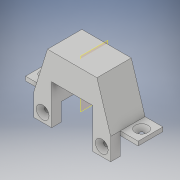
# Autodesk Inventor part: buttonHolder
Saved by Autodesk Inventor 2019 (Build 230136000, 136)
## iProperties
Created: 2019-08-23
Part Number: buttonHolder
Material: Generic
Document SubType Name: Modeling
Designer: fablab
Density: 1 g/cm^3
Appearance: Default
Author: fablab
Autodesk Inventor part; units mm, degrees
ref_plane "YZ Plane" through (0, 0, 0) normal (1, 0, 0) x (0, 1, 0)
ref_plane "XZ Plane" through (0, 0, 0) normal (0, 1, 0) x (-1, 0, 0)
ref_plane "XY Plane" through (0, 0, 0) normal (0, 0, 1) x (1, 0, 0)
sketch "Sketch1" plane through (0, 0, 0) normal (0, 1, 0) x (-1, 0, 0)
  line L0 (0, 0) -> (-30, 0)
  line L1 (-30, 0) -> (-30, -10.6)
  line L2 (-30, -10.6) -> (0, -10.6)
  line L3 (0, -10.6) -> (0, 0)
  line L4 (0, -10.6) -> (1.1, -10.6)
  line L5 (1.1, -10.6) -> (1.1, -18)
  line L6 (1.1, -18) -> (0, -18)
  line L7 (0, -18) -> (0, -10.6)
  line L8 (-30, -10.6) -> (-31.1, -10.6)
  line L9 (-31.1, -10.6) -> (-31.1, -18)
  line L10 (-31.1, -18) -> (-30, -18)
  line L11 (-30, -18) -> (-30, -10.6)
  line L12 (0, -18) -> (-30, -18)
  dimension "d0" = 30
  dimension "d1" = 10.6
  dimension "d2" = 1.1
  dimension "d3" = 1.1
  dimension "d4" = 7.4
  dimension "d5" = 7.4
  constraints: 26 end point, 6 parallel, 3 horizontal, 3 perpendicular
  measures "d0" distance of L2.end L1.end
  measures "d1" distance of L1.end L0.end
  measures "d2" distance of L5.end L6.end
  measures "d3" distance of L10.end L9.end
  measures "d4" distance of L8.end L9.end
  measures "d5" distance of L4.end L5.end
extrude "Extrusion1" add sketch "Sketch1" along normal blind 3
sketch "Sketch2" plane through (30, 0, 0) normal (1, 0, 0) x (0, 0, -1)
  point P0 (0, 0)
sketch "Sketch3" plane through (30, 0, 0) normal (1, 0, 0) x (0, 0, -1)
  line L0 (0, 0) -> (10.6, 0) projected
  line L1 (0, 0) -> (0, -30)
  line L2 (0, -30) -> (10.6, -30)
  line L3 (10.6, 0) -> (10.6, -30)
  line L4 (10.6, 0) -> (0, 0) projected
  line L5 (0, 0) -> (10.6, 0)
  dimension "d8" = 30
  constraints: 8 end point, 2 vertical, 1 collinear, 1 perpendicular
  measures "d8" distance of L0.start L1.end
sketch "Sketch4" plane through (31.1, 0, -10.6) normal (1, 0, 0) x (0, 0, -1)
  line L0 (0, 0) -> (7.4, 0) projected
  line L1 (7.4, 0) -> (7.4, -14)
  line L2 (7.4, -14) -> (0, -14)
  line L3 (0, -14) -> (0, 0)
  line L4 (0, 0) -> (7.4, 0)
  point P0 (-10.6, 0)
  dimension "d9" = 14
  constraints: 8 end point, 2 perpendicular, 1 collinear, 1 vertical
  measures "d9" distance of L0.end L1.end
extrude "Extrusion2" add sketch "Sketch3" along normal blind 3
extrude "Extrusion3" add sketch "Sketch4" along normal blind 3
sketch "Sketch5" plane through (31.1, -14, -18) normal (0, -1, 0) x (1, 0, 0)
  line L0 (1.9, 7.4) -> (1.9, 18) projected
  line L1 (1.9, 7.4) -> (1.9, 0)
  line L2 (0, 0) -> (3, 0) projected
  line L3 (-1.1, 18) -> (-1.1, 7.4) projected
  line L4 (-1.1, 7.4) -> (-1.1, 0)
  line L5 (0, 0) -> (-32.2, 0) projected
  line L6 (-1.1, 7.4) -> (1.9, 7.4) projected
  line L7 (1.9, 7.4) -> (-1.1, 7.4)
  point P0 (-31.1, 18)
  constraints: 6 end point, 2 point on line, 1 horizontal, 1 parallel, 1 vertical
extrude "Extrusion4" add sketch "Sketch5" along normal blind 16
sketch "Sketch6" plane through (30, 0, 0) normal (0, 1, 0) x (1, 0, 0)
  line L0 (1.1, 10.6) -> (1.1, 18) projected
  line L1 (1.1, 10.6) -> (1.1, 0)
  line L2 (0, 0) -> (3, 0) projected
  line L3 (1.1, 0) -> (0, 0)
  line L4 (0, 0) -> (0, 10.6)
  line L5 (0, 0) -> (0, 18) projected
  line L6 (0, 10.6) -> (1.1, 10.6) projected
  line L7 (1.1, 10.6) -> (0, 10.6)
  point P0 (-30, 0)
  constraints: 8 end point, 2 collinear, 1 point on line, 1 vertical
extrude "Extrusion5" add sketch "Sketch6" along normal blind 3
sketch "Sketch7" plane through (31.1, 3, 0) normal (1, 0, 0) x (0, 0, -1)
  point P0 (0, -3)
sketch "Sketch8" plane through (31.1, 0, 0) normal (0, 1, 0) x (1, 0, 0)
  line L0 (0, 0) -> (1.9, 0) projected
  line L1 (0, 0) -> (0, 18) projected
  line L2 (1.9, 0) -> (0, 0)
  line L3 (0, 0) -> (0, 18)
  line L4 (0, 18) -> (1.9, 18)
  line L5 (1.9, 18) -> (1.9, 0)
  point P0 (-31.1, 0)
  constraints: 8 end point, 2 parallel, 1 horizontal, 1 perpendicular
extrude "Extrusion6" add sketch "Sketch8" along normal up to surface (3 mm away)
sketch "Sketch9" plane through (33, -14, -10.6) normal (0, 0, 1) x (1, 0, 0)
  line L0 (0, 0) -> (0, 14) projected
  line L1 (0, 0) -> (1.1, 0) projected
  line L2 (1.1, 14) -> (1.1, 0) projected
  line L3 (0, 14) -> (1.1, 14) projected
  line L4 (0, 0) -> (0, 14) projected
  line L5 (0, 14) -> (1.1, 14)
  line L6 (1.1, 14) -> (1.1, 0)
  line L7 (1.1, 0) -> (0, 0)
  line L8 (0, 0) -> (0, 14)
  point P0 (-33, 14)
  constraints: 8 end point, 2 parallel, 1 horizontal, 1 perpendicular
extrude "Extrusion7" cut sketch "Sketch9" against normal blind 2000
sketch "Sketch10" plane through (33, 0, 0) normal (1, 0, 0) x (0, 0, -1)
  line L0 (0, -30) -> (0, 3) projected
  line L1 (0, -30) -> (18, -30)
  line L2 (18, -30) -> (18, -27)
  line L3 (18, -27) -> (0, -27)
  line L4 (0, -27) -> (0, -30)
  point P0 (0, 0)
  point P1 (0, 1.1)
  dimension "d25" = 18
  dimension "d26" = 3
  constraints: 8 end point, 2 parallel, 1 horizontal, 1 perpendicular
  measures "d25" distance of L3.end L2.end
  measures "d26" distance of L2.end L1.end
extrude "Extrusion8" add sketch "Sketch10" along normal blind 14
sketch "Sketch12" plane through (0, 3, 0) normal (0, 1, 0) x (1, 0, 0)
  line L0 (0, 10.6) -> (0, 0) projected
  line L1 (15, 0) -> (15, 18)
  point P0 (30, 10.6)
  point P1 (31.1, 10.6)
  point P2 (30, 0)
  constraints: 2 end point, 1 vertical
ref_plane "Work Plane1" through (15, 0, -10.6) normal (-1, 0, 0) x (0, 0, 1)
mirror "Mirror1" about plane through (15, 0, -10.6) normal (-1, 0, 0) of "Extrusion2", "Extrusion3", "Extrusion4", "Extrusion5", "Extrusion6", "Extrusion7", "Extrusion8"
sketch "Sketch13" plane through (30, -30, 0) normal (0, 0, 1) x (1, 0, 0)
  line L0 (-33, 33) -> (3, 33) projected
  line L1 (-30, 30) -> (0, 30)
  line L2 (0, 30) -> (0, 33)
  line L3 (0, 33) -> (-30, 33)
  line L4 (-30, 33) -> (-30, 30)
  point P0 (-31.1, 33)
  point P1 (1.1, 33)
  dimension "d36" = 30
  constraints: 8 end point, 2 parallel, 1 horizontal, 1 perpendicular, 1 point on line
  measures "d36" distance of L3.end L2.end
extrude "Extrusion10" add sketch "Sketch13" along normal blind 7
sketch "Sketch14" plane through (0, 0, 0) normal (0, -1, 0) x (1, 0, 0)
  line L0 (0, 0) -> (0, 7) projected
  line L1 (30, 0) -> (30, -10.6) projected
  line L2 (0, 7) -> (30, 7)
  line L3 (30, 7) -> (30, 0)
  line L4 (30, 0) -> (0, 0)
  line L5 (0, 0) -> (0, 7)
  constraints: 8 end point, 2 parallel, 1 horizontal, 1 perpendicular
extrude "Extrusion11" add sketch "Sketch14" along normal blind 14
sketch "Sketch16" plane through (0, 3, 0) normal (0, 1, 0) x (1, 0, 0)
  line L0 (30, -7) -> (0, -7) projected
  line L1 (-3, 18) -> (33, 18) projected
  line L2 (30, -7) -> (0, -7)
  line L3 (0, -7) -> (0, 18)
  line L4 (0, 18) -> (30, 18)
  line L5 (30, 18) -> (30, -7)
  line L6 (33, 18) -> (31.1, 18) projected
  line L7 (31.1, 18) -> (30, 18)
  line L8 (30, 18) -> (30, 0)
  line L9 (30, 0) -> (31.1, 0)
  line L10 (0, 0) -> (0, 18) projected
  line L11 (0, 18) -> (-1.1, 18)
  line L12 (-1.1, 0) -> (0, 0)
  line L13 (0, 0) -> (0, 18)
  line L14 (31.1, 18) -> (33, 18)
  line L15 (33, 0) -> (31.1, 0)
  line L16 (33, 0) -> (30, 0) projected
  line L17 (31.1, 18) -> (-1.1, 18) projected
  line L18 (-3, 18) -> (-17, 18) projected
  line L19 (-1.1, 18) -> (-3, 18)
  line L20 (-3, 18) -> (-3, 0) projected
  line L21 (-3, 18) -> (-3, 0)
  line L22 (-3, 0) -> (-1.1, 0)
  line L23 (0, 0) -> (-3, 0) projected
  line L24 (33, 18) -> (33, 0) projected
  line L25 (33, 18) -> (33, 0)
  constraints: 32 end point, 5 collinear, 4 horizontal, 4 parallel, 2 perpendicular, 1 point on line
extrude "Extrusion13" add sketch "Sketch16" along normal blind 2
sketch "Sketch17" plane through (30, -30, 0) normal (0, 0, 1) x (1, 0, 0)
  line L0 (0, 35) -> (3, 35) projected
  line L1 (3, 35) -> (0, 35)
  line L2 (0, 35) -> (0, 0)
  line L3 (0, 0) -> (3, 0)
  line L4 (3, 0) -> (3, 35)
  line L5 (0, 0) -> (17, 0) projected
  line L6 (0, 0) -> (13, 0)
  line L7 (13, 0) -> (13, -13.0001)
  line L8 (13, -13.0001) -> (0, -13.0001)
  line L9 (0, -13.0001) -> (0, 0)
  point P0 (-30, 30)
  dimension "d45" = 13
  constraints: 16 end point, 4 parallel, 2 horizontal, 2 perpendicular
  measures "d45" distance of L7.end L8.end
extrude "Extrusion14" add sketch "Sketch17" along normal blind 7 contours L0 L4 L3 L2
sketch "Sketch18" plane through (33, -30, 0) normal (0, 0, 1) x (1, 0, 0)
  line L0 (-3, 16) -> (-3, 0) projected
  line L1 (-3, 0) -> (10, 0)
  line L2 (10, 0) -> (10, -13)
  line L3 (10, -13) -> (-3, -13)
  line L4 (-3, -13) -> (-3, 0)
  point P0 (-33, 30)
  dimension "d48" = 13
  dimension "d49" = 13
  constraints: 8 end point, 2 parallel, 1 horizontal, 1 perpendicular
  measures "d48" distance of L2.end L3.end
  measures "d49" distance of L1.end L2.end
extrude "Extrusion15" add sketch "Sketch18" along normal blind 7
sketch "Sketch19" plane through (33, -30, 0) normal (0, 1, 0) x (1, 0, 0)
  line L0 (10, 0) -> (10, -7) projected
  line L1 (10, -7) -> (0, -7) projected
  line L2 (10, 0) -> (0, 0)
  line L3 (0, 0) -> (0, -7)
  line L4 (0, -7) -> (10, -7)
  line L5 (10, -7) -> (10, 0)
  point P0 (-33, 0)
  constraints: 8 end point, 2 parallel, 1 horizontal, 1 perpendicular
sketch "Sketch20" plane through (30, -30, 7) normal (0, 0, 1) x (1, 0, 0)
  line L0 (13, -13) -> (13, 0) projected
  line L1 (13, -6.5) -> (0, -6.5) construction
  line L2 (0, -13) -> (0, 0) projected
  line L3 (3, 0) -> (13, 0) projected
  line L4 (6.5, 0) -> (6.5, -6.5) construction
  circle A0 centre (6.5, -6.5) radius 1.65
  point P0 (-30, 30)
  dimension "d52" = 3.3
  constraints: 4 end point, 3 midpoint, 1 centre point, 1 coincident, 1 point on line
  measures "d52" diameter of A0
extrude "Extrusion16" cut sketch "Sketch20" against normal blind 7
chamfer "Chamfer3" distance 3 angle 45 1 edges at (34.85, -36.5, 7)
extrude "Extrusion17" add sketch "Sketch19" along normal blind 3
sketch "Sketch21" plane through (33, -27, -18) normal (0, 1, 0) x (1, 0, 0)
  line L0 (14, 0) -> (14, -18) projected
  line L1 (14, 0) -> (23, 0)
  line L2 (23, 0) -> (23, -18)
  line L3 (23, -18) -> (14, -18)
  line L4 (14, -18) -> (14, 0)
  point P0 (-33, -18)
  dimension "d60" = 9
  constraints: 8 end point, 2 parallel, 1 horizontal, 1 perpendicular
  measures "d60" distance of L2.end L3.end
extrude "Extrusion18" add sketch "Sketch21" against normal blind 3
sketch "Sketch22" plane through (33, -27, 7) normal (0, 1, 0) x (1, 0, 0)
  line L0 (10, 7) -> (23, 7) projected
  line L1 (16.5, 7) -> (16.5, 25) construction
  line L2 (0, 25) -> (23, 25) projected
  line L3 (23, 25) -> (23, 7) projected
  line L4 (23, 16) -> (16.5, 16) construction
  circle A0 centre (16.5, 16) radius 1.65
  point P0 (-33, 7)
  dimension "d63" = 3.3
  constraints: 4 end point, 3 midpoint, 1 centre point, 1 coincident, 1 point on line, 1 vertical
  measures "d63" diameter of A0
extrude "Extrusion19" cut sketch "Sketch22" against normal blind 3
chamfer "Chamfer4" distance 3 angle 45 1 edges at (47.85, -27, -9)
sketch "Sketch24" plane through (30, -30, 7) normal (0, 0, 1) x (1, 0, 0)
  line L0 (1.1, 30) -> (1.1, 16) projected
  line L1 (-30, 35) -> (3, 35) projected
  line L2 (-30, 16) -> (-30, 35) projected
  line L3 (0, 16) -> (-30, 16) projected
  line L4 (0, 16) -> (0, -13) projected
  line L5 (0, -13) -> (13, -13) projected
  line L6 (13, -13) -> (13, 3) projected
  line L7 (3, 3) -> (13, 3) projected
  line L8 (3, 3) -> (3, 35) projected
  circle A0 centre (6.5, -6.5) radius 4.65 projected
  line L9 (3, 35) -> (3, 3) projected
  line L10 (3, 35) -> (3, 3)
  line L11 (3, 3) -> (13, 3)
  line L12 (3, 35) -> (13, 3)
  point P0 (-30, 30)
  constraints: 6 end point, 2 collinear
extrude "Extrusion20" add sketch "Sketch24" against normal blind 25 contours L12 L7 L8
ref_plane "Work Plane2" through (15, 0, 0) normal (1, 0, 0) x (0, 0, -1)
mirror "Mirror2" about plane through (15, 0, 0) normal (1, 0, 0) of "Extrusion1", "Extrusion2", "Extrusion3", "Extrusion4", "Extrusion5", "Extrusion6", "Extrusion7", "Extrusion8", "Extrusion10", "Extrusion11", "Extrusion13", "Extrusion14", "Extrusion15", "Extrusion16", "Chamfer3", "Extrusion17", "Extrusion18", "Extrusion19", "Chamfer4", "Extrusion20"
ref_plane "Work Plane3" through (15, 0, -10.6) normal (-1, 0, 0) x (0, 0, 1)
body "Solid1"
